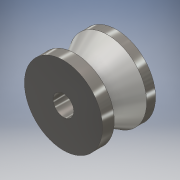
# Autodesk Inventor part: Peça 9
Saved by Autodesk Inventor 2016 (Build 200138000, 138)
## iProperties
Created: 2018-09-28
Part Number: Peça 9
Material: Generic
Document SubType Name: Sheet Metal
Designer: dqm_r
Density: 1 g/cm^3
Appearance: Default
Sheet Metal Rule: Default
Author: dqm_r
Autodesk Inventor part; units mm, degrees
ref_plane "YZ Plane" through (0, 0, 0) normal (1, 0, 0) x (0, 1, 0)
sketch "Sketch1" plane through (0, 0, 0) normal (0, 1, 0) x (-1, 0, 0)
  circle A0 centre (0, 0) radius 7
  dimension "d0" = 14
  constraints: 1 centre point, 1 coincident
  measures "d0" diameter of A0
extrude "Extrusion1" add sketch "Sketch1" along normal blind 2.12
sketch "Sketch3" plane through (0, 2.12, 0) normal (0, 1, 0) x (1, 0, 0)
  circle A0 centre (0, 0) radius 4.5
  dimension "d4" = 9
  constraints: 1 centre point, 1 coincident
  measures "d4" diameter of A0
extrude "Extrusion2" add sketch "Sketch3" along normal blind 1.3
ref_plane "Work Plane2" through (0, 7.92, 0) normal (0, 1, 0) x (1, 0, 0)
sketch "Sketch5" plane through (0, 7.92, 0) normal (0, 1, 0) x (1, 0, 0)
  circle A0 centre (0, 0) radius 7
  dimension "d8" = 14
  constraints: 1 centre point, 1 coincident
  measures "d8" diameter of A0
loft "Loft1" add profiles "Sketch5" section 1 edges at (-4.5, 3.42, 0)
sketch "Sketch7" plane through (0, 7.92, 0) normal (0, 1, 0) x (1, 0, 0)
  circle A0 centre (0, 0) radius 7
  constraints: 1 centre point, 1 coincident
extrude "Extrusion3" add sketch "Sketch7" along normal blind 1.6
sketch "Sketch8" plane through (0, 9.52, 0) normal (0, 1, 0) x (1, 0, 0)
  circle A0 centre (0, 0) radius 5.2
  dimension "d15" = 10.4
  constraints: 1 centre point, 1 coincident
  measures "d15" diameter of A0
ref_plane "Work Plane3" through (0, 3.42, 0) normal (0, 1, 0) x (1, 0, 0)
sketch "Sketch10" plane through (0, 3.42, 0) normal (0, 1, 0) x (1, 0, 0)
  circle A0 centre (0, 0) radius 1.85
  dimension "d22" = 3.7
  constraints: 1 centre point, 1 coincident
  measures "d22" diameter of A0
loft "Loft3" cut profiles "Sketch8", "Sketch10"
hole "Hole1" at (0, 0, 0) direction (0, 1, 0) diameter 3.7 end through all
equation "\"d34\" = Thickness"
equation "\"BendRadius\" = Thickness"
equation "\"BendReliefWidth\" = Thickness"
equation "\"BendReliefDepth\" = 0.5 * Thickness"
equation "\"CornerReliefSize\" = 4 * Thickness"
equation "\"MinimumRemnant\" = 2 * Thickness"
equation "\"TransitionRadius\" = BendRadius"
equation "\"JacobiRadiusSize\" = Thickness"
equation "\"GapSize\" = Thickness"
equation "\"Thickness\" = 0.5"
body "Solid1"
